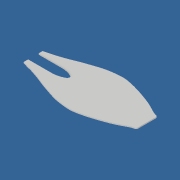
# Autodesk Inventor part: Part2
Saved by Autodesk Inventor 2018 (Build 220112000, 112)
## iProperties
Created: 2018-03-02
Part Number: Part2
Material: Generic
Document SubType Name: Modeling
Designer: 232963
Density: 1 g/cm^3
Appearance: Default
Author: 232963
Autodesk Inventor part; units mm, degrees
ref_plane "YZ Plane" through (0, 0, 0) normal (1, 0, 0) x (0, 1, 0)
ref_plane "XZ Plane" through (0, 0, 0) normal (0, 1, 0) x (-1, 0, 0)
ref_plane "XY Plane" through (0, 0, 0) normal (0, 0, 1) x (1, 0, 0)
sketch "Sketch1" plane through (0, 0, 0) normal (0, 0, 1) x (1, 0, 0)
  line L0 (-34.346, 0) -> (308.554, 0)
  line L1 (-34.346, 2.794) -> (-34.346, 0)
  line L2 (-34.346, 2.794) -> (308.554, 2.794)
  line L3 (308.554, 2.794) -> (308.554, 0)
  point P0 (0, 0)
  dimension "d102" = 342.9
  constraints: 8 end point, 1 horizontal, 1 vertical, 1 other
  measures "d102" distance from line of L0.end L1
extrude "Extrusion1" add sketch "Sketch1" along normal blind 161.925
sketch "Sketch2" plane through (-34.346, 2.794, 0) normal (0, 1, 0) x (1, 0, 0)
  line L0 (0, 0) -> (0, -161.925) projected
  line L1 (0, -80.9625) -> (355.6, -80.9625)
  line L2 (342.9, 0) -> (0, 0) projected
  line L3 (0, 0) -> (342.9, 0) projected
  spline S0 degree 4 poles (190.5, 0) (176.6775, 0) (146.1194, -4.9047) (146.8521, -3.1203) (83.6356, -24.6252) (79.4605, -26.74) (68.0118, -31.1235) (63.3839, -33.2828) (38.0924, -42.0424) (22.0487, -47.0453) (18.7736, -46.718) (0.7177, -52.7069) (0, -52.4002) knots 0 0 0 0 0 0.204521 0.323697 0.422378 0.506708 0.581474 0.662125 0.742434 0.828574 1 1 1 1 1
  line L4 (0, -52.4002) -> (0, 0)
  line L5 (190.5, 0) -> (0, 0)
  line L6 (342.9, 0) -> (342.9, -161.925) projected
  spline S1 degree 4 poles (190.5, 0) (208.4411, 0) (251.3479, -12.7353) (261.4383, -16.5213) (279.9875, -22.867) (307.7965, -33.882) (329.1012, -47.2629) (336.8853, -48.836) (342.9, -49.53) knots 0 0 0 0 0 0.297202 0.471636 0.622976 0.773941 1 1 1 1 1
  line L7 (324.9507, -47.459) -> (360.8493, -51.601) construction
  arc A0 (328.7385, -47.0401) -> (357.2564, -50.3305) centre (356.8343, 71.2391) ccw construction
  line L8 (199.9843, 0) -> (190.5, 0)
  point P0 (34.346, 0)
  point P1 (0, -112.0775)
  point P2 (184.15, -161.925)
  point P3 (6.35, -50.8)
  point P4 (19.05, -47.244)
  point P5 (25.4, -45.72)
  point P6 (63.5, -33.02)
  point P7 (38.1, -41.91)
  point P8 (76.2, -27.94)
  point P9 (127, -10.16)
  point P10 (152.4, -3.81)
  point P11 (69.85, -30.48)
  point P12 (82.55, -25.4)
  point P13 (266.7, -18.288)
  point P14 (279.4, -22.86)
  point P15 (304.8, -33.655)
  point P16 (330.2, -46.355)
  point P17 (342.9, -49.53)
  dimension "d8" = 31.115
  dimension "d9" = 184.15
  dimension "d12" = 52.4002
  dimension "d13" = 50.8
  dimension "d15" = 47.244
  dimension "d16" = 6.35
  dimension "d19" = 6.35
  dimension "d20" = 45.72
  dimension "d31" = 41.91
  dimension "d35" = 33.02
  dimension "d37" = 27.94
  dimension "d38" = 12.7
  dimension "d45" = 10.16
  dimension "d49" = 3.81
  dimension "d57" = 30.48
  dimension "d58" = 6.35
  dimension "d60" = 25.4
  dimension "d89" = 190.5
  dimension "d95" = 12.7
  dimension "d96" = 12.7
  dimension "d107" = 13.97
  dimension "d108" = 18.288
  dimension "d109" = 22.86
  dimension "d111" = 33.655
  dimension "d112" = 46.355
  dimension "d113" = 25.4
  dimension "d114" = 49.53
  constraints: 10 end point, 5 point on line, 3 collinear, 3 midpoint, 2 horizontal, 1 centre point, 1 point on circle, 21 other
  measures "d8" distance of point (0, -112.078) L1.start
  measures "d9" distance of L0.end point (184.15, -161.925)
  measures "d12" distance from line of L2 L4.start
  measures "d13" distance from line of L2 point (6.35, -50.8)
  measures "d15" distance from line of L2 point (19.05, -47.244)
  measures "d16" horizontal distance of point (6.35, -50.8) L4.start
  measures "d19" horizontal distance of point (25.4, -45.72) point (19.05, -47.244)
  measures "d20" distance from line of L2 point (25.4, -45.72)
  measures "d31" distance from line of L2 point (38.1, -41.91)
  measures "d35" distance from line of L2 point (63.5, -33.02)
  measures "d37" distance from line of L2 point (76.2, -27.94)
  measures "d38" horizontal distance of point (63.5, -33.02) point (76.2, -27.94)
  measures "d45" distance from line of L2 point (127, -10.16)
  measures "d49" distance from line of L2 point (152.4, -3.81)
  measures "d57" distance from line of L2 point (69.85, -30.48)
  measures "d58" horizontal distance of point (76.2, -27.94) point (69.85, -30.48)
  measures "d60" distance from line of L2 point (82.55, -25.4)
  measures "d89" horizontal distance of L5.start L4.start
  measures "d95" horizontal distance of point (266.7, -18.288) point (254, -13.97)
  measures "d96" horizontal distance of point (279.4, -22.86) point (266.7, -18.288)
  measures "d107" distance from line of L2 point (254, -13.97)
  measures "d108" distance from line of L2 point (266.7, -18.288)
  measures "d109" distance from line of L2 point (279.4, -22.86)
  measures "d111" distance from line of L2 point (304.8, -33.655)
  measures "d112" distance from line of L2 point (330.2, -46.355)
  measures "d113" horizontal distance of point (304.8, -33.655) point (330.2, -46.355)
  measures "d114" distance from line of point (342.9, -49.53) L2
extrude "Extrusion2" cut sketch "Sketch2" against normal blind 25.4 contours L2 S0 L0 | L2 L6 S1
ref_plane "Work Plane2" through (0, 0, 80.9625) normal (0, 0, -1) x (-1, 0, 0)
mirror "Mirror1" about plane through (0, 0, 80.9625) normal (0, 0, -1) of "Extrusion2"
sketch "Sketch3" plane through (308.554, 2.794, 161.925) normal (0, 1, 0) x (1, 0, 0)
  line L0 (-342.9, 109.5248) -> (-342.9, 52.4002) projected
  line L1 (-342.9, 97.6249) -> (-273.05, 97.6249)
  line L2 (-234.95, 96.0374) -> (-234.95, 9.9368) construction
  line L3 (-273.05, 65.8749) -> (-342.9, 65.8749)
  line L4 (-342.9, 65.8749) -> (-342.9, 97.6249)
  line L5 (-273.05, 97.6249) -> (-273.05, 65.8749)
  arc A0 (-273.05, 65.8749) -> (-238.76, 74.1299) centre (-273.05, 141.2201) ccw
  arc A1 (-238.76, 89.3699) -> (-273.05, 97.6249) centre (-273.05, 22.2797) ccw
  line L6 (-238.76, 96.0374) -> (-238.76, 64.2874) construction
  spline S0 degree 4 poles (-238.76, 74.1299) (-236.6016, 75.2331) (-232.3793, 77.6246) (-232.3793, 85.8752) (-236.6016, 88.2667) (-238.76, 89.3699) knots 0 0 0 0 0 0.5 1 1 1 1 1
  point P0 (-308.554, 161.925)
  dimension "d75" = 31.75
  dimension "d78" = 57.1246
  dimension "d79" = 11.8999
  dimension "d80" = 38.1
  dimension "d81" = 15.24
  dimension "d82" = 0
  dimension "d83" = 8.255
  dimension "d84" = 3.81
  dimension "d85" = 0
  dimension "d86" = 107.95
  constraints: 12 end point, 4 point on circle, 2 centre point, 2 parallel, 2 perpendicular, 2 tangent, 1 horizontal, 1 point on line, 1 vertical, 4 other
  measures "d75" distance between parallel lines of L3 L1
  measures "d78" distance of L0.end L0.start
  measures "d79" distance of L0.start L1.start
  measures "d80" distance between parallel lines of L2 L5
  measures "d81" distance of A0.end A1.start
  measures "d82" horizontal distance of A0.end A1.start
  measures "d83" distance from line of A0.end L3
  measures "d84" distance between parallel lines of L6 L2
  measures "d85" distance from line of L6 A1.start
  measures "d86" distance from line of L2 L3.end
extrude "Extrusion3" cut sketch "Sketch3" against normal blind 25.4
fillet "Fillet1" radius 5.715 1 edges at (308.554, 1.397, 49.53)
fillet "Fillet2" radius 5.715 1 edges at (308.554, 1.397, 112.395)
equation "\"d8\" = d7"
equation "\"d7\" = 31.115"
body "Solid1"
